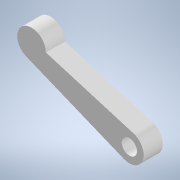
# Autodesk Inventor part: Palanca metacarpo_distal
Saved by Autodesk Inventor 2020.4 (Build 244396010, 396A)
## iProperties
Created: 2021-08-20
Part Number: Palanca metacarpo_distal
Material: Generic
Document SubType Name: Modeling
Designer: chalo
Density: 1 g/cm^3
Appearance: Default
Author: chalo
Autodesk Inventor part; units mm, degrees
ref_plane "YZ Plane" through (0, 0, 0) normal (1, 0, 0) x (0, 1, 0)
ref_plane "XZ Plane" through (0, 0, 0) normal (0, 1, 0) x (-1, 0, 0)
ref_plane "XY Plane" through (0, 0, 0) normal (0, 0, 1) x (1, 0, 0)
sketch "Sketch1" plane through (0, 0, 0) normal (0, 0, 1) x (1, 0, 0)
  circle A0 centre (91.35, 6.3991) radius 1.6 projected
  circle A1 centre (70.85, 18.1613) radius 2.25
  circle A2 centre (91.35, 6.3991) radius 3
  line L0 (76.4305, 15.9113) -> (89.3317, 4.1796)
  line L1 (78.8117, 18.6299) -> (93.0461, 8.8737)
  circle A3 centre (70.85, 13.6613) radius 1.6 projected
  circle A4 centre (70.85, 18.1613) radius 1.625 projected
  line L2 (76.4305, 15.9113) -> (70.85, 15.9113)
  line L3 (78.8117, 18.6299) -> (72.5761, 19.6046)
  point P0 (0, 0)
  point P1 (72.1824, 12.7754)
  point P2 (69.5176, 12.7754)
  dimension "d0" = 4.5
  dimension "d1" = 6
  constraints: 8 end point, 4 point on circle, 3 tangent, 2 centre point, 2 coincident
  measures "d0" diameter of A1
  measures "d1" diameter of A2
extrude "Extrusion1" add sketch "Sketch1" along normal mid plane 4 contours A1 | A1 L3 L1 A2 L0 L2 | A2
body "Solid1"
